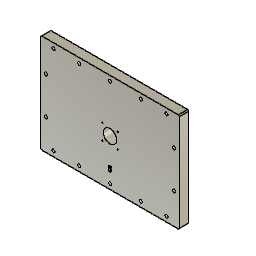
CAD_File 7 (Autodesk Fusion 360 design; units mm, degrees)
Autodesk Fusion 360 part; units mm, degrees
sketch "Sketch1" plane through (0, 115, 0) normal (0, 1, 0) x (-1, 0, 0)
  line L0 (-115, -20) -> (-135, -20)
  line L1 (-135, -20) -> (-135, -172.35)
  line L2 (-135, -172.35) -> (-115, -172.35)
  line L3 (-115, -172.35) -> (-115, -20)
  line L4 (-135, 0) -> (-135, -20)
  line L5 (-135, -20) -> (-135, -172.35)
  line L6 (-135, -172.35) -> (-135, -192.35)
  line L7 (135, -192.35) -> (-135, -192.35)
  line L8 (135, -20) -> (135, -172.35)
  line L9 (135, -172.35) -> (135, -192.35)
  line L10 (135, 0) -> (135, -20)
  line L11 (135, 0) -> (-135, 0)
extrude "Extrude1" add sketch "Sketch1" along normal blind 20
sketch "Sketch2" plane through (0, 135, 0) normal (0, 1, 0) x (-1, 0, 0)
  line L0 (-135, 0) -> (-135, -192.35)
  circle A0 centre (0, -102.55) radius 13
  circle A1 centre (-15, -87.55) radius 1.5
  circle A2 centre (15, -87.55) radius 1.5
  circle A3 centre (15, -117.55) radius 1.5
  circle A4 centre (-15, -117.55) radius 1.5
  line L1 (135, -192.35) -> (135, 0)
  line L2 (135, 0) -> (-135, 0)
  line L3 (-135, -192.35) -> (135, -192.35)
  dimension "d520" = 3
  dimension "d521" = 3
  dimension "d522" = 3
  dimension "d523" = 3
  dimension "d524" = 26
  dimension "d525" = 15
  dimension "d526" = 15
  dimension "d527" = 30
  dimension "d528" = 30
  dimension "d529" = 30
  measures "d520" diameter of A2
  measures "d521" diameter of A3
  measures "d522" diameter of A4
  measures "d523" diameter of A1
  measures "d524" diameter of A0
  measures "d525" horizontal distance of A0.centre A2.centre
  measures "d526" vertical distance of A0.centre A2.centre
  measures "d527" distance of A1.centre A2.centre
  measures "d528" distance of A1.centre A4.centre
  measures "d529" distance of A3.centre A4.centre
extrude "Extrude2" cut sketch "Sketch2" against normal up to surface (20 mm away) contours A0 | A1 | A2 | A3 | A4
thread "Thread1" "ANSI Unified Screw Threads 0.112(#4) 4-40 UNC 3B" major diameter 2.8448 minor diameter 2.2708 pitch 0.635 angle 60 resizes the face on face at (13.5905, 121.6667, -87.037) on face at (-16.4095, 121.6667, -87.037) on face at (-16.4095, 121.6667, -117.037) on face at (13.5905, 121.6667, -117.037)
chamfer "Chamfer1" distance 2 angle 45 8 edges at (-135, 125, 0) (-135, 135, -96.175) (0, 135, 0) (0, 135, -192.35) (-135, 125, -192.35) (135, 125, -192.35) (135, 125, 0) (135, 135, -96.175)
sketch "Sketch3" plane through (0, 135, 0) normal (0, 1, 0) x (-1, 0, 0)
  circle A0 centre (-15, -117.55) radius 1.1354
  circle A1 centre (0, -102.55) radius 13
  circle A2 centre (15, -117.55) radius 1.1354
  circle A3 centre (-15, -87.55) radius 1.1354
  circle A4 centre (15, -87.55) radius 1.1354
  line L0 (-133, -2) -> (-133, -190.35)
  line L1 (-133, -190.35) -> (133, -190.35)
  line L2 (133, -190.35) -> (133, -2)
  line L3 (133, -2) -> (-133, -2)
  line L4 (0, 10) -> (0, -200) construction
  line L5 (-150, -96.175) -> (150, -96.175) construction
  circle A5 centre (-110, -10) radius 3
  circle A6 centre (0, -10) radius 3
  line L6 (133, 0) -> (-133, 0)
  line L7 (-135, -2) -> (-135, -190.35)
  circle A7 centre (-110, -10) radius 5.5
  circle A8 centre (0, -10) radius 5.5
  circle A9 centre (-125, -60) radius 3
  circle A10 centre (-60, -10) radius 3
  circle A11 centre (-125, -60) radius 5.5
  circle A12 centre (125, -60) radius 3
  circle A13 centre (125, -60) radius 5.5
  circle A14 centre (110, -10) radius 5.5
  circle A15 centre (110, -10) radius 3
  circle A16 centre (60, -10) radius 3
  circle A17 centre (-125, -132.35) radius 5.5
  circle A18 centre (-125, -132.35) radius 3
  circle A19 centre (-110, -182.35) radius 5.5
  circle A20 centre (-110, -182.35) radius 3
  circle A21 centre (-60, -182.35) radius 3
  circle A22 centre (0, -182.35) radius 5.5
  circle A23 centre (0, -182.35) radius 3
  circle A24 centre (60, -182.35) radius 3
  circle A25 centre (110, -182.35) radius 5.5
  circle A26 centre (110, -182.35) radius 3
  circle A27 centre (125, -132.35) radius 5.5
  circle A28 centre (125, -132.35) radius 3
  dimension "d574" = 94.175
  dimension "d575" = 94.175
  dimension "d576" = 6
  dimension "d577" = 6
  dimension "d579" = 10
  dimension "d581" = 10
  dimension "d582" = 25
  dimension "d584" = 11
  dimension "d585" = 11
  dimension "d586" = 6
  dimension "d591" = 10
  dimension "d592" = 60
  dimension "d594" = 6
  dimension "d595" = 10
  dimension "d596" = 75
  dimension "d597" = 11
  constraint perpendicular L1 L4
  constraint perpendicular L2 L5
  constraint coincident L4 A6.centre
  constraint concentric A5 A7
  constraint concentric A6 A8
  constraint concentric A9 A11
  constraint symmetric L4 A5 A15
  constraint symmetric L4 A7 A14
  constraint symmetric L4 A9 A12
  constraint symmetric L4 A10 A16
  constraint symmetric L4 A11 A13
  constraint symmetric L5 A5 A20
  constraint symmetric L5 A6 A23
  constraint symmetric L5 A7 A19
  constraint symmetric L5 A8 A22
  constraint symmetric L5 A9 A18
  constraint symmetric L5 A10 A21
  constraint symmetric L5 A11 A17
  constraint symmetric L5 A12 A28
  constraint symmetric L5 A13 A27
  constraint symmetric L5 A14 A25
  constraint symmetric L5 A15 A26
  constraint symmetric L5 A16 A24
  measures "d574" distance of L2.end L5
  measures "d575" distance of L1.end L5
  measures "d576" diameter of A5
  measures "d577" diameter of A6
  measures "d579" distance of A5.centre L6
  measures "d581" distance of A6.centre L6
  measures "d582" distance of A5.centre L7
  measures "d584" diameter of A7
  measures "d585" diameter of A8
  measures "d586" diameter of A9
  measures "d591" distance of L7 A9.centre
  measures "d592" distance of L6 A9.centre
  measures "d594" diameter of A10
  measures "d595" distance of L6 A10.centre
  measures "d596" horizontal distance of L7.start A10.centre
  measures "d597" diameter of A11
extrude "Extrude3" cut sketch "Sketch3" against normal blind 40 contours A5 | A6 | A9 | A12 | A15 | A18 | A20 | A23 | A26 | A28
extrude "Extrude4" cut sketch "Sketch3" against normal blind 35 contours A10 | A16 | A21 | A24
extrude "Extrude5" cut sketch "Sketch3" against normal blind 6.5 contours A7 | A8 | A11 | A13 | A14 | A17 | A19 | A22 | A25 | A27
sketch "Sketch4" plane through (0, 115, 0) normal (0, -1, 0) x (1, 0, 0)
  circle A0 centre (-60, -182.35) radius 3
  circle A1 centre (60, -10) radius 3
  circle A2 centre (60, -182.35) radius 3
  circle A3 centre (-60, -10) radius 3
  circle A4 centre (0, -182.35) radius 3
  circle A5 centre (-110, -10) radius 3
  circle A6 centre (125, -60) radius 3
  circle A7 centre (-125, -60) radius 3
  circle A8 centre (110, -182.35) radius 3
  circle A9 centre (-110, -182.35) radius 3
  circle A10 centre (0, -10) radius 3
  circle A11 centre (110, -10) radius 3
  circle A12 centre (-125, -132.35) radius 3
  circle A13 centre (125, -132.35) radius 3
  line L0 (133, -192.35) -> (135, -190.35)
  line L1 (135, -190.35) -> (135, -2)
  line L2 (135, -2) -> (133, 0)
  line L3 (133, 0) -> (-133, 0)
  line L4 (-133, 0) -> (-135, -2)
  line L5 (-135, -2) -> (-135, -190.35)
  line L6 (-135, -190.35) -> (-133, -192.35)
  line L7 (-133, -192.35) -> (133, -192.35)
  circle A14 centre (-15, -87.55) radius 1.1354
  circle A15 centre (15, -87.55) radius 1.1354
  circle A16 centre (-15, -117.55) radius 1.1354
  circle A17 centre (0, -102.55) radius 13
  circle A18 centre (15, -117.55) radius 1.1354
  line L8 (-3.4202, -160.0273) -> (-2.131, -159.9181)
  spline S0 degree 2 poles (-2.131, -159.9181) (-1.9877, -160.8595) (-1.4659, -161.3336) knots 0 0 0 1 1 1
  spline S1 degree 2 poles (-1.4659, -161.3336) (-0.9441, -161.8076) (-0.2074, -161.8076) knots 0 0 0 1 1 1
  spline S2 degree 2 poles (-0.2074, -161.8076) (0.6794, -161.8076) (1.2933, -161.1392) knots 0 0 0 1 1 1
  spline S3 degree 2 poles (1.2933, -161.1392) (1.9072, -160.4707) (1.9072, -159.3656) knots 0 0 0 1 1 1
  spline S4 degree 2 poles (1.9072, -159.3656) (1.9072, -158.3151) (1.3172, -157.7081) knots 0 0 0 1 1 1
  spline S5 degree 2 poles (1.3172, -157.7081) (0.7271, -157.101) (-0.2278, -157.101) knots 0 0 0 1 1 1
  spline S6 degree 2 poles (-0.2278, -157.101) (-0.8213, -157.101) (-1.2988, -157.3704) knots 0 0 0 1 1 1
  spline S7 degree 2 poles (-1.2988, -157.3704) (-1.7763, -157.6398) (-2.0491, -158.0696) knots 0 0 0 1 1 1
  line L9 (-2.0491, -158.0696) -> (-3.2019, -157.9195)
  line L10 (-3.2019, -157.9195) -> (-2.2333, -152.7831)
  line L11 (-2.2333, -152.7831) -> (2.7394, -152.7831)
  line L12 (2.7394, -152.7831) -> (2.7394, -153.9563)
  line L13 (2.7394, -153.9563) -> (-1.251, -153.9563)
  line L14 (-1.251, -153.9563) -> (-1.7899, -156.6439)
  spline S8 degree 2 poles (-1.7899, -156.6439) (-0.8895, -156.0164) (0.0996, -156.0164) knots 0 0 0 1 1 1
  spline S9 degree 2 poles (0.0996, -156.0164) (1.4093, -156.0164) (2.3097, -156.9236) knots 0 0 0 1 1 1
  spline S10 degree 2 poles (2.3097, -156.9236) (3.2101, -157.8308) (3.2101, -159.2565) knots 0 0 0 1 1 1
  spline S11 degree 2 poles (3.2101, -159.2565) (3.2101, -160.6139) (2.4188, -161.603) knots 0 0 0 1 1 1
  spline S12 degree 2 poles (2.4188, -161.603) (1.457, -162.8172) (-0.2074, -162.8172) knots 0 0 0 1 1 1
  spline S13 degree 2 poles (-0.2074, -162.8172) (-1.5716, -162.8172) (-2.4345, -162.0532) knots 0 0 0 1 1 1
  spline S14 degree 2 poles (-2.4345, -162.0532) (-3.2974, -161.2892) (-3.4202, -160.0273) knots 0 0 0 1 1 1
extrude "Extrude6" cut sketch "Sketch4" against normal blind 0.2 contours L8 S0 S1 S2 S3 S4 S5 S6 S7 L9 L10 L11 L12 L13 L14 S8 S9 S10 S11 S12 S13 S14
